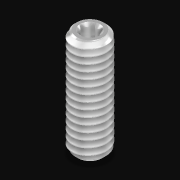
# Autodesk Inventor part: Coupler Star 1
Saved by Autodesk Inventor 2021 (Build 250183000, 183)
## iProperties
Created: 2020-07-03
Part Number: Coupler Star 1
Material: VEX Steel
Document SubType Name: Modeling
Designer: yuany
Density: 1 g/cm^3
Appearance: Screws
Author: yuany
Autodesk Inventor part; units mm, degrees
ref_plane "YZ Plane" through (0, 0, 0) normal (1, 0, 0) x (0, 1, 0)
ref_plane "XZ Plane" through (0, 0, 0) normal (0, 1, 0) x (-1, 0, 0)
ref_plane "XY Plane" through (0, 0, 0) normal (0, 0, 1) x (1, 0, 0)
sketch "Sketch1" plane through (0, 0, 0) normal (0, 1, 0) x (-1, 0, 0)
  circle A0 centre (0, 0) radius 1.5621
  dimension "d4" = 3.1242
  constraints: 1 centre point, 1 coincident
  measures "d4" diameter of A0
extrude "Body" add sketch "Sketch1" along normal blind 12.7
sketch "Sketch5" plane through (0, 0, 0) normal (1, 0, 0) x (0, 1, 0)
  line L0 (0, -1.5621) -> (12.7, -1.5621)
  line L1 (0.07452, -1.5621) -> (-0.226106, -2.0828)
  line L2 (-0.226106, -2.0828) -> (-0.325325, -2.0828)
  line L3 (-0.325325, -2.0828) -> (-0.625951, -1.5621)
  line L4 (0.06858, -2.0828) -> (-0.72517, -2.0828) construction
  line L5 (-0.625951, -1.5621) -> (0.07452, -1.5621)
  line L6 (0, -1.5621) -> (12.7, -1.5621)
  line L7 (12.7, -1.5621) -> (12.7, 1.5621)
  point P0 (0, 0)
  dimension "d32" = 60
  dimension "a" = 0.09922
  dimension "d46" = 0.79375
  dimension "d54" = 0.06858
  dimension "d55" = 0.5207
  dimension "d56" = 0.09922
  dimension "d57" = 30
  constraints: 10 end point, 2 collinear, 2 point on line, 1 horizontal
  measures "d32" angle of L1 L3
  measures "a" distance of L1.end L2.end
  measures "d46" distance of L4.start L4.end
  measures "d54" horizontal distance of L4.start L6.start
  measures "d55" distance between parallel lines of L2 L5
  measures "d56" horizontal distance of L3.end L4.end
  measures "d57" angle of L1 L7
coil "Thread" sketch "Sketch5" operation add axis through (0, -10, 0) along (0, 1, 0) pitch 0.79375 turns 17.6 hand right
sketch "Sketch6" plane through (0, 0, 0) normal (0, 0, 1) x (1, 0, 0)
  line L0 (0, 0) -> (-1.4859, 0)
  line L1 (1.516382, 0) -> (0, 0)
  line L2 (-1.4859, 0) -> (-2.494763, 1.008863)
  line L3 (-2.494763, 1.008863) -> (-2.965078, -1.218824)
  line L4 (-2.965078, -1.218824) -> (-1.4859, -1.218824)
  line L5 (-1.5621, 0.272958) -> (-1.5621, 12.272486)
  line L6 (-1.4859, -1.218824) -> (-1.4859, 0)
  line L7 (0, -6.457086) -> (0, 30.210748)
  point P0 (0, 0)
  point P1 (-2.0828, 0.5969)
  dimension "d49" = 1.4859
  dimension "d50" = 135
  constraints: 10 end point, 1 horizontal, 1 vertical, 3 other
  measures "d49" distance from line of L0.start L6
  measures "d50" angle of L2 L6
revolve "Tapered End" cut sketch "Sketch6" angle 360 about axis through (0, -10, 0) along (0, 1, 0)
sketch "Sketch7" plane through (0, 12.7, 0) normal (0, 1, 0) x (1, 0, 0)
  circle A0 centre (0, 0) radius 2.663263
  constraints: 1 centre point, 1 coincident
extrude "Flatten Threads" cut sketch "Sketch7" along normal blind 12.7
sketch "Sketch8" plane through (0, 12.7, 0) normal (0, 1, 0) x (1, 0, 0)
  line L0 (-1.1938, 0.689241) -> (0, 1.378482)
  line L1 (0, 1.378482) -> (1.1938, 0.689241)
  line L2 (1.1938, 0.689241) -> (1.1938, -0.689241)
  line L3 (1.1938, -0.689241) -> (0, -1.378482)
  line L4 (0, -1.378482) -> (-1.1938, -0.689241)
  line L5 (-1.1938, -0.689241) -> (-1.1938, 0.689241)
  point P0 (0, 0)
  point P1 (0, 0)
  dimension "d60" = 2.3876
  constraints: 12 end point, 1 coincident, 1 vertical, 13 other
  measures "d60" distance between parallel lines of L2 L5
extrude "Hex" [suppressed]
sketch "Sketch9" plane through (0, 0, 0) normal (0, 0, 1) x (1, 0, 0)
  line L0 (1.1938, 11.5824) -> (0.5588, 11.2014)
  line L1 (0.5588, 11.2014) -> (0, 11.2014)
  line L2 (0, 11.2014) -> (0, 11.5824)
  line L3 (0, 11.5824) -> (1.1938, 11.5824)
  point P0 (0, 0)
  dimension "d104" = 0.381
  dimension "d105" = 0.5588
  dimension "d106" = 1.1938
  dimension "d107" = 0
  dimension "d108" = 11.5824
  constraints: 9 end point, 2 horizontal, 1 perpendicular
  measures "d104" distance of L1.end L2.end
  measures "d105" distance of L0.end L1.end
  measures "d106" distance of L2.end L0.start
  measures "d107" distance from line of point (0, 0) L2
  measures "d108" distance from line of point (0, 0) L3
revolve "Hex Divot" [suppressed]
sketch "Sketch10" plane through (0, 0, 0) normal (0, 0, 1) x (1, 0, 0)
  line L0 (0, 10.765712) -> (-1.1938, 11.2014)
  line L1 (-1.1938, 11.2014) -> (-1.1938, 12.7)
  line L2 (-1.1938, 12.7) -> (0, 12.7)
  line L3 (0, 12.7) -> (0, 10.765712)
  line L4 (0, -5.08) -> (0, 30.48)
  line L5 (-1.4859, 0) -> (1.4859, 0)
  point P0 (0, 0)
  dimension "d70" = 20.05
  dimension "d71" = 1.1938
  dimension "d73" = 1.4986
  dimension "d75" = 12.7
  constraints: 8 end point, 1 collinear, 1 perpendicular, 1 vertical
  measures "d70" angle of L2 L0
  measures "d71" distance of L1.end L2.end
  measures "d73" distance of L0.end L1.end
  measures "d75" distance between parallel lines of L5 L2
revolve "Star" cut sketch "Sketch10" angle 360 about axis through (0, -10, 0) along (0, 1, 0)
sketch "Sketch11" plane through (0, 12.7, 0) normal (0, 1, 0) x (1, 0, 0)
  arc A0 (-0.5969, -0.769897) -> (-0.3683, -0.901879) centre (-0.5207, -0.901879) ccw
  arc A1 (-0.670859, -0.875838) -> (-1.093927, -0.143062) centre (-1.321547, -0.762995) ccw
  line L0 (-1.0414, 0) -> (-0.5207, 0.901879) construction
  line L1 (-0.5207, 0.901879) -> (0.5207, 0.901879) construction
  line L2 (0.5207, 0.901879) -> (1.0414, 0) construction
  line L3 (1.0414, 0) -> (0.5207, -0.901879) construction
  line L4 (0.5207, -0.901879) -> (-0.5207, -0.901879) construction
  line L5 (-0.5207, -0.901879) -> (-1.0414, 0) construction
  arc A2 (0.5969, 0.769897) -> (0.3683, 0.901879) centre (0.5207, 0.901879) ccw
  arc A3 (-0.3683, 0.901879) -> (-0.5969, 0.769897) centre (-0.5207, 0.901879) ccw
  arc A4 (0.9652, -0.131982) -> (0.9652, 0.131982) centre (1.0414, 0) ccw
  arc A5 (0.3683, -0.901879) -> (0.5969, -0.769897) centre (0.5207, -0.901879) ccw
  arc A6 (-0.9652, 0.131982) -> (-0.9652, -0.131982) centre (-1.0414, 0) ccw
  arc A7 (-1.093927, 0.143062) -> (-0.670859, 0.875838) centre (-1.321547, 0.762995) ccw
  arc A8 (-0.423069, 1.0189) -> (0.423069, 1.0189) centre (0, 1.525991) ccw
  arc A9 (0.670859, 0.875838) -> (1.093927, 0.143062) centre (1.321547, 0.762995) ccw
  arc A10 (1.093927, -0.143062) -> (0.670859, -0.875838) centre (1.321547, -0.762995) ccw
  arc A11 (0.423069, -1.0189) -> (-0.423069, -1.0189) centre (0, -1.525991) ccw
  circle A12 centre (0, 0) radius 1.271513
  dimension "d76" = 0.3048
  dimension "d77" = 2.0828
  dimension "d78" = 1.3208
  dimension "d79" = 0.3048
  dimension "d80" = 0.3048
  dimension "d81" = 0.3048
  dimension "d82" = 0.3048
  dimension "d83" = 0.3048
  dimension "d84" = 1.3208
  dimension "d85" = 1.3208
  dimension "d86" = 1.3208
  dimension "d87" = 1.3208
  dimension "d88" = 1.3208
  constraints: 36 point on circle, 13 centre point, 12 end point, 12 point on line, 12 tangent, 8 coincident, 1 horizontal, 13 other
  measures "d76" diameter of A0
  measures "d77" distance of L0.start L2.end
  measures "d78" diameter of A1
  measures "d79" diameter of A2
  measures "d80" diameter of A3
  measures "d81" diameter of A4
  measures "d82" diameter of A5
  measures "d83" diameter of A6
  measures "d84" diameter of A7
  measures "d85" diameter of A8
  measures "d86" diameter of A9
  measures "d87" diameter of A10
  measures "d88" diameter of A11
extrude "Star 2" add sketch "Sketch11" against normal blind 6.35
sketch "Sketch12" plane through (0, 0, 0) normal (0, 0, 1) x (1, 0, 0)
  line L0 (-1.1938, 12.7) -> (0, 12.7)
  line L1 (0, 12.7) -> (0, 11.5062)
  line L2 (0, 11.5062) -> (-1.1938, 12.7)
  line L3 (0, -5.08) -> (0, 30.48) projected
  point P0 (0, 0)
  dimension "d91" = 45
  dimension "d93" = 12.7
  dimension "d94" = 0
  dimension "d95" = 1.1938
  constraints: 6 end point, 1 horizontal, 1 vertical
  measures "d91" angle of L0 L2
  measures "d93" distance from line of point (0, 0) L0
  measures "d94" horizontal distance of point (0, 0) L0.end
  measures "d95" distance of L0.start L0.end
revolve "Star 3" cut sketch "Sketch12" angle 360 about axis through (0, -10, 0) along (0, 1, 0)
sketch "Sketch13" plane through (0, 0, 0) normal (0, 0, 1) x (1, 0, 0)
  line L0 (0, 12.7) -> (-1.5748, 12.7)
  line L1 (-1.5748, 12.7) -> (-2.842327, 11.432473)
  line L2 (-2.842327, 11.432473) -> (-2.842327, 12.7)
  line L3 (-2.842327, 12.7) -> (-1.5748, 12.7)
  line L4 (0, -5.08) -> (0, 30.48)
  point P0 (0, 0)
  dimension "d109" = 45
  dimension "d110" = 0
  dimension "d111" = 1.5748
  dimension "d112" = 12.7
  constraints: 8 end point, 1 collinear, 1 horizontal, 1 point on line, 1 vertical
  measures "d109" angle of L3 L1
  measures "d110" horizontal distance of point (0, 0) L0.start
  measures "d111" distance of L0.start L0.end
  measures "d112" distance from line of point (0, 0) L0
revolve "Tapered Head" cut sketch "Sketch13" angle 360 about axis through (0, -10, 0) along (0, 1, 0)
equation "\"d56\" = a"
body "Solid1"
